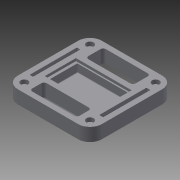
# Autodesk Inventor part: 14 pin long holder
Saved by Autodesk Inventor 2015 (Build 190159000, 159)
## iProperties
Created: 2014-12-11
Part Number: 14 pin long holder
Material: Generic
Document SubType Name: Modeling
Designer: Purple
Density: 1 g/cm^3
Appearance: Default
Author: Purple
Autodesk Inventor part; units mm, degrees
ref_plane "YZ Plane" through (0, 0, 0) normal (1, 0, 0) x (0, 1, 0)
ref_plane "XZ Plane" through (0, 0, 0) normal (0, 1, 0) x (-1, 0, 0)
sketch "Sketch1" plane through (0, 0, 0) normal (0, 1, 0) x (-1, 0, 0)
  line L0 (30, 30) -> (-30, 30)
  line L1 (-30, 30) -> (-30, -30)
  line L2 (-30, -30) -> (30, -30)
  line L3 (30, -30) -> (30, 30)
  line L4 (30, 30) -> (-30, -30) construction
  line L5 (-30, 30) -> (30, -30) construction
  point P0 (0, 0)
  dimension "d0" = 60
  dimension "d1" = 60
  constraints: 12 end point, 2 midpoint, 2 parallel, 1 horizontal, 1 perpendicular
  measures "d0" distance of L2.end L1.end
  measures "d1" distance of L0.end L1.end
extrude "Extrusion1" add sketch "Sketch1" along normal blind 10
fillet "Fillet1" radius 7 4 edges at (30, 5, 30) (30, 5, -30) (-30, 5, 30) (-30, 5, -30)
sketch "Sketch2" plane through (0, 10, 0) normal (0, 1, 0) x (1, 0, 0)
  line L0 (-30, 30) -> (30, 30)
  line L1 (30, 30) -> (30, -30)
  line L2 (30, -30) -> (-30, -30)
  line L3 (-30, -30) -> (-30, 30)
  line L4 (-30, 30) -> (30, -30) construction
  line L5 (30, 30) -> (-30, -30) construction
  line L6 (25, -25) -> (25, 25)
  line L7 (25, 25) -> (-25, 25)
  line L8 (-25, 25) -> (-25, -25)
  line L9 (-25, -25) -> (25, -25)
  circle A0 centre (25, -25) radius 2.75
  circle A1 centre (-25, -25) radius 2.75
  circle A2 centre (25, 25) radius 2.75
  circle A3 centre (-25, 25) radius 2.75
  point P0 (0, 0)
  dimension "d5" = 5
  dimension "d6" = 5.5
  dimension "d7" = 5.5
  dimension "d8" = 5.5
  dimension "d9" = 5.5
  constraints: 20 end point, 4 centre point, 4 coincident, 4 parallel, 2 midpoint, 2 perpendicular, 1 horizontal, 3 other
  measures "d5" distance between parallel lines of L1 L6
  measures "d6" diameter of A0
  measures "d7" diameter of A1
  measures "d8" diameter of A2
  measures "d9" diameter of A3
extrude "Extrusion2" cut sketch "Sketch2" against normal blind 3 contours L9 A0 L6 | L6 A0 L9 | A2 L7 L6 | L6 L7 A2 | A1 L8 L9 | L9 L8 A1 | A3 L8 L7 | L7 L8 A3
sketch "Sketch7" plane through (0, 10, 0) normal (0, 1, 0) x (1, 0, 0)
  line L0 (-23, 30) -> (23, 30)
  line L1 (30, 23) -> (30, -23)
  line L2 (23, -30) -> (-23, -30)
  line L3 (-30, -23) -> (-30, 23)
  line L4 (-30, 30) -> (30, -30) construction
  line L5 (30, 30) -> (-30, -30) construction
  arc A0 (-23, 30) -> (-30, 23) centre (-23, 23) ccw
  arc A1 (-30, -23) -> (-23, -30) centre (-23, -23) ccw
  arc A2 (23, -30) -> (30, -23) centre (23, -23) ccw
  arc A3 (30, 23) -> (23, 30) centre (23, 23) ccw
  line L6 (23, 32) -> (-23, 32)
  arc A4 (-23, 32) -> (-32, 23) centre (-23, 23) ccw
  line L7 (-32, 23) -> (-32, -23)
  arc A5 (-32, -23) -> (-23, -32) centre (-23, -23) ccw
  line L8 (-23, -32) -> (23, -32)
  arc A6 (23, -32) -> (32, -23) centre (23, -23) ccw
  line L9 (32, -23) -> (32, 23)
  arc A7 (32, 23) -> (23, 32) centre (23, 23) ccw
  point P0 (0, 0)
  dimension "d47" = 7
  dimension "d48" = 2
  constraints: 20 end point, 16 point on circle, 8 centre point, 8 point on line, 8 tangent, 4 parallel, 3 equal radius, 2 midpoint, 2 perpendicular, 1 horizontal, 7 other
  measures "d47" radius of A0
  measures "d48" distance between parallel lines of L0 L6
extrude "Extrusion6" add sketch "Sketch7" against normal blind 10
sketch "Sketch17" plane through (0, 10, 0) normal (0, 1, 0) x (1, 0, 0)
  circle A0 centre (25, -25) radius 2.75 projected
  line L0 (-25, 25) -> (25, 25)
  line L1 (25, 25) -> (25, -25)
  line L2 (25, -25) -> (-25, -25)
  line L3 (-25, -25) -> (-25, 25)
  line L4 (-25, 25) -> (25, -25) construction
  line L5 (25, 25) -> (-25, -25) construction
  line L6 (21, -21) -> (21, 10.7)
  line L7 (-21.4, -13) -> (21, -13)
  line L8 (21, 10.7) -> (-21.4, 10.7)
  line L9 (-21.4, -13) -> (-21.4, 10.7)
  line L10 (-19.4, 9.7) -> (-19.4, -11)
  line L11 (-19.4, -11) -> (19, -11)
  line L12 (19, 9.7) -> (-19.4, 9.7)
  line L13 (19, 9.7) -> (19, -11)
  point P0 (0, 0)
  dimension "d134" = 50
  dimension "d135" = 50
  dimension "d136" = 4
  dimension "d137" = 8
  dimension "d138" = 42.4
  dimension "d139" = 23.7
  dimension "d141" = 1
  dimension "d142" = 2
  constraints: 28 end point, 4 perpendicular, 2 midpoint, 2 parallel, 1 horizontal, 1 point on line
  measures "d134" distance of L1.end L2.end
  measures "d135" distance of L0.end L1.end
  measures "d136" distance between parallel lines of L1 L6
  measures "d137" distance of L7.end L6.start
  measures "d138" distance of L7.start L7.end
  measures "d139" distance of L6.end L7.end
  measures "d141" distance between parallel lines of L8 L12
  measures "d142" distance from line of L12.start L6
extrude "Extrusion15" cut sketch "Sketch17" against normal blind 2 contours L7 L9 L8 L6
sketch "Sketch18" plane through (0, 10, 0) normal (0, 1, 0) x (1, 0, 0)
  line L0 (-19.4, 9.7) -> (19, 9.7)
  line L1 (19, 9.7) -> (19, -11)
  line L2 (19, -11) -> (-19.4, -11)
  line L3 (-19.4, -11) -> (-19.4, 9.7)
  point P0 (0, 0)
  constraints: 8 end point, 2 parallel, 1 horizontal, 1 perpendicular
extrude "Extrusion16" cut sketch "Sketch18" against normal blind 8
sketch "Sketch19" plane through (0, 10, 0) normal (0, 1, 0) x (1, 0, 0)
  line L0 (23, 32) -> (-23, 32) projected
  line L1 (-32, 23) -> (-32, -23) projected
  line L2 (32, -23) -> (32, 23) projected
  line L3 (-21.4, 10.7) -> (21, 10.7) projected
  line L4 (-18, 14.7) -> (-18, 28)
  line L5 (-18, 28) -> (18, 28)
  line L6 (18, 28) -> (18, 14.7)
  line L7 (18, 14.7) -> (-18, 14.7)
  line L8 (-23, -32) -> (23, -32) projected
  line L9 (-28, -18) -> (-28, 18)
  line L10 (-21.4, -13) -> (-21.4, 10.7) projected
  line L11 (-28, -18) -> (-25.4, -18)
  line L12 (-25.4, -18) -> (-25.4, 18)
  line L13 (-25.4, 18) -> (-28, 18)
  line L14 (21, 10.7) -> (21, -13) projected
  line L15 (28, 18) -> (25, 18)
  line L16 (25, 18) -> (25, -18)
  line L17 (25, -18) -> (28, -18)
  line L18 (28, -18) -> (28, 18)
  line L19 (21, -13) -> (-21.4, -13) projected
  line L20 (18, -28) -> (18, -17)
  line L21 (18, -28) -> (-18, -28)
  line L22 (-18, -28) -> (-18, -17)
  line L23 (-18, -17) -> (18, -17)
  point P0 (0, 0)
  dimension "d147" = 4
  dimension "d148" = 14
  dimension "d149" = 4
  dimension "d150" = 14
  dimension "d151" = 4
  dimension "d152" = 4
  dimension "d153" = 4
  dimension "d154" = 4
  dimension "d155" = 14
  dimension "d156" = 14
  dimension "d157" = 4
  dimension "d158" = 4
  dimension "d159" = 14
  dimension "d160" = 4
  dimension "d161" = 14
  dimension "d162" = 4
  dimension "d163" = 4
  dimension "d164" = 4
  dimension "d165" = 14
  dimension "d166" = 14
  dimension "d167" = 4
  constraints: 32 end point, 7 perpendicular, 2 horizontal, 2 vertical
  measures "d147" distance from line of L4.end L0
  measures "d148" distance from line of L1 L4.end
  measures "d149" distance from line of L5.end L0
  measures "d150" distance from line of L2 L5.end
  measures "d151" distance from line of L6.end L3
  measures "d152" distance from line of L3 L4.start
  measures "d153" distance from line of L1 L9.start
  measures "d154" distance from line of L1 L9.end
  measures "d155" distance from line of L9.start L8
  measures "d156" distance from line of L0 L9.end
  measures "d157" distance from line of L11.end L10
  measures "d158" distance from line of L2 L15.start
  measures "d159" distance from line of L0 L15.start
  measures "d160" distance from line of L2 L17.end
  measures "d161" distance from line of L8 L17.end
  measures "d162" distance from line of L15.end L14
  measures "d163" distance from line of L8 L20.start
  measures "d164" distance from line of L8 L21.end
  measures "d165" distance from line of L2 L20.start
  measures "d166" distance from line of L1 L21.end
  measures "d167" distance from line of L20.end L19
extrude "Extrusion17" cut sketch "Sketch19" against normal through all contours L4 L5 L6 L7 | L9 L13 L12 L11 | L18 L17 L16 L15 | L21 L22 L23 L20
fillet "Fillet5" radius 2 8 edges at (18, 5, -28) (18, 5, 17) (-18, 5, -28) (-18, 5, 17) (-18, 5, -14.7) (-18, 5, 28) (18, 5, -14.7) (18, 5, 28)
fillet "Fillet5" radius 0.5 12 edges at (28, 5, 18) (-25.4, 5, 18) (28, 5, -18) (-25.4, 5, -18) (-28, 5, -18) (25, 5, -18) (-0.2, 2, -9.7) (-19.4, 2, 0.65) (-0.2, 2, 11) (-28, 5, 18) (25, 5, 18) (19, 2, 0.65)
ref_plane "Work Plane4" through (0, 5, 0) normal (0, 1, 0) x (1, 0, 0)
mirror "Mirror4" about plane through (0, 5, 0) normal (0, 1, 0) of "Extrusion2"
body "Solid1"
